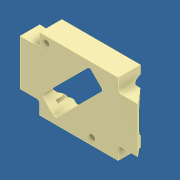
# Autodesk Inventor part: GuideCarotte
Saved by Autodesk Inventor 2018 (Build 220112000, 112)
## iProperties
Created: 2022-03-08
Part Number: GuideCarotte
Material: Nylon 6/6
Document SubType Name: Modeling
Designer: Nathann
Density: 1.13 g/cm^3
Appearance: Nylon 6
Mass: 63.4787 g
Surface Area: 154.903 cm^2
Volume: 56.1759 cm^3
Author: Nathann
Autodesk Inventor part; units mm, degrees
ref_plane "YZ Plane" through (0, 0, 0) normal (1, 0, 0) x (0, 1, 0)
ref_plane "XZ Plane" through (0, 0, 0) normal (0, 1, 0) x (-1, 0, 0)
sketch "Sketch24" plane through (0, 0, 0) normal (0, 1, 0) x (-1, 0, 0)
  line L0 (0, 0) -> (90, 0)
  line L1 (90, 0) -> (90, 55)
  line L2 (90, 55) -> (0, 55)
  line L3 (0, 55) -> (0, 0)
  dimension "d160" = 55
  dimension "d161" = 90
  constraints: 8 end point, 2 parallel, 1 horizontal, 1 perpendicular
  measures "d160" distance of L0.end L1.end
  measures "d161" distance of L1.end L2.end
extrude "Extrusion21" add sketch "Sketch24" along normal blind 17
sketch "Sketch25" plane through (0, 0, 0) normal (0, -1, 0) x (1, 0, 0)
  circle A0 centre (-70, 50) radius 2.5
  circle A1 centre (-35, 5) radius 2.5
  line L0 (0, 0) -> (-90, 0) projected
  line L1 (-90, 55) -> (0, 55) projected
  line L2 (-90, 0) -> (-90, 55) projected
  dimension "d164" = 5
  dimension "d165" = 5
  dimension "d166" = 5
  dimension "d167" = 5
  dimension "d168" = 20
  dimension "d169" = 55
  constraints: 2 centre point
  measures "d164" diameter of A0
  measures "d165" diameter of A1
  measures "d166" distance from line of L0 A1.centre
  measures "d167" distance from line of L1 A0.centre
  measures "d168" distance from line of L2 A0.centre
  measures "d169" distance from line of L2 A1.centre
extrude "Extrusion22" cut sketch "Sketch25" against normal blind 14
sketch "Sketch26" plane through (0, 17, 0) normal (0, 1, 0) x (1, 0, 0)
  line L0 (-63.0815, -3.8119) -> (-26.3119, -40.5815)
  line L1 (-26.3119, -40.5815) -> (-36.9185, -51.1881)
  line L2 (-36.9185, -51.1881) -> (-73.6881, -14.4185)
  line L3 (-73.6881, -14.4185) -> (-63.0815, -3.8119)
  line L4 (-90, 0) -> (-90, -55) projected
  line L5 (0, 0) -> (-90, 0) projected
  point P0 (0, -22.5)
  dimension "d172" = 15
  dimension "d173" = 52
  dimension "d176" = 47.3762
  dimension "d177" = 47.3762
  dimension "d181" = 16.3119
  dimension "d182" = 45
  dimension "d183" = 3.8119
  constraints: 8 end point, 3 perpendicular
  measures "d172" distance of L0.end L1.end
  measures "d173" distance of L1.end L2.end
  measures "d176" horizontal distance of L2.end L0.end
  measures "d177" vertical distance of L1.end L0.start
  measures "d181" distance from line of L4 L2.end
  measures "d182" angle of L4 L2
  measures "d183" distance from line of L5 L0.start
extrude "Extrusion23" cut sketch "Sketch26" against normal through all
ref_plane "Work Plane2" through (0, 0, 55) normal (0.9994, 0, 0.0349) x (0, 1, 0)
sketch "Sketch28" plane through (0, 0, 55) normal (0.9994, 0, 0.0349) x (0, 1, 0)
  circle A0 centre (27, -25.9665) radius 22.5
  line L0 (17, 0) -> (17, -54.9665) projected
  line L1 (0, -54.9665) -> (17, -54.9665) projected
  line L2 (0, 0) -> (0, -54.9665) projected
  dimension "d187" = 45
  dimension "d192" = 29
  dimension "d194" = 27
  constraints: 1 centre point
  measures "d187" diameter of A0
  measures "d192" distance from line of A0.centre L1
  measures "d194" distance from line of L2 A0.centre
extrude "Extrusion24" cut sketch "Sketch28" against normal through all
sketch "Sketch29" plane through (0, 17, 0) normal (0, 1, 0) x (1, 0, 0)
  line L0 (-26.3119, -40.5815) -> (-63.0815, -3.8119) projected
  line L1 (-44.6967, -22.1967) -> (-55.3033, -32.8033)
  line L2 (-73.6881, -14.4185) -> (-40.3293, -47.7773) projected
  arc A0 (-68.4344, -7.51) -> (-69.99, -9.0656) centre (-70.0818, -7.4182) ccw
  line L3 (-63.5547, -12.3896) -> (-68.4344, -7.51)
  line L4 (-69.99, -9.0656) -> (-65.1104, -13.9453)
  line L5 (-65.1104, -13.9453) -> (-63.5547, -12.3896)
  line L6 (-65.8208, -6.5512) -> (-63.0815, -3.8119) projected
  arc A1 (-31.5656, -47.49) -> (-30.01, -45.9344) centre (-29.9182, -47.5818) ccw
  line L7 (-34.8896, -41.0547) -> (-30.01, -45.9344)
  line L8 (-31.5656, -47.49) -> (-36.4453, -42.6104)
  line L9 (-36.4453, -42.6104) -> (-34.8896, -41.0547)
  line L10 (-29.0512, -43.3208) -> (-26.3119, -40.5815)
  point P0 (0, 0)
  point P1 (-73.6881, -14.4185)
  point P2 (-56.553, -49.6596)
  point P3 (-21.3119, -14.4185)
  point P4 (-40.3293, -47.7773)
  point P5 (-36.9185, -51.1881)
  dimension "d216" = 2.2
  dimension "d217" = 1.1
  dimension "d218" = 3.3
  dimension "d219" = 2.4
  dimension "d221" = 7.5
  dimension "d222" = 15
  constraints: 16 end point, 7 symmetric about line, 4 point on circle, 2 centre point, 1 midpoint, 1 parallel, 1 perpendicular, 3 other
  measures "d216" distance of L4.end L3.start
  measures "d217" distance from line of L3 A0.centre
  measures "d218" diameter of A0
  measures "d219" distance from line of A0.centre L6
  measures "d221" distance from line of A0.centre L0
extrude "Extrusion25" cut sketch "Sketch29" against normal blind 10.5
fillet "Fillet4" radius 2 4 edges at (-26.3119, 4.1375, 40.5815) (-63.0815, 8.5, 3.8119) (-73.6881, 3.9894, 14.4185) (-36.9185, 8.5, 51.1881)
sketch "Sketch31" plane through (0, 0, 0) normal (0, -1, 0) x (1, 0, 0)
  line L0 (7.4187, -6.4354) -> (-15, -6.4354)
  line L1 (-15, -6.4354) -> (-15, 10)
  line L2 (-15, 10) -> (7.4187, 10)
  line L3 (7.4187, 10) -> (7.4187, -6.4354)
  line L4 (0, 55) -> (0, 0) projected
  line L5 (0, 0) -> (-90, 0) projected
  line L6 (0, 0) -> (-90, 0) projected
  line L7 (-90, 55) -> (0, 55) projected
  line L8 (0, 27.5) -> (-90, 27.5)
  line L9 (-45, 62.4242) -> (-45, -8.4375)
  line L10 (-90, 0) -> (-90, 55) projected
  line L11 (7.4187, 61.4354) -> (-15, 61.4354)
  line L12 (-15, 61.4354) -> (-15, 45)
  line L13 (-15, 45) -> (7.4187, 45)
  line L14 (7.4187, 45) -> (7.4187, 61.4354)
  line L15 (-97.4187, -6.4354) -> (-75, -6.4354)
  line L16 (-75, -6.4354) -> (-75, 10)
  line L17 (-75, 10) -> (-97.4187, 10)
  line L18 (-97.4187, 10) -> (-97.4187, -6.4354)
  line L19 (-90, 55) -> (-90, 0)
  line L20 (-97.4187, 61.4354) -> (-75, 61.4354)
  line L21 (-75, 61.4354) -> (-75, 45)
  line L22 (-75, 45) -> (-97.4187, 45)
  line L23 (-97.4187, 45) -> (-97.4187, 61.4354)
  point P0 (-17, 0)
  point P1 (-17, 55)
  point P2 (-73, 0)
  point P3 (-73, 55)
  dimension "d227" = 15
  dimension "d228" = 10
  dimension "d229" = 45
  dimension "d230" = 90
  constraints: 38 end point, 14 symmetric about line, 3 perpendicular, 2 horizontal, 2 parallel, 1 midpoint, 1 vertical
  measures "d227" distance between parallel lines of L1 L4
  measures "d228" distance between parallel lines of L2 L5
  measures "d229" distance between parallel lines of L10 L9
  measures "d230" distance between parallel lines of L10 L4
extrude "Extrusion27" cut sketch "Sketch31" against normal through all contours L0 L1 L5 L4 L2 L3 | L1 L2 L4 L5 | L16 L15 L18 L17 L10 L5 | L5 L10 L17 L16 | L13 L12 L7 L4 | L4 L7 L12 L11 L14 L13 | L22 L23 L20 L21 L7 L10 | L10 L7 L21 L22
fillet "Fillet5" radius 2 4 edges at (-15, 7.0843, 10) (-75, 5.7918, 10) (-75, 7.1624, 45) (-15, 5.8494, 45)
sketch "Sketch32" plane through (0, 0, 45) normal (0, 0, 1) x (1, 0, 0)
  line L0 (0, 0) -> (-24.7878, 29.541)
  line L1 (-24.7878, 29.541) -> (8.6873, 22.432)
  line L2 (8.6873, 22.432) -> (0, 0)
  line L3 (0, 0) -> (-13, 0) projected
  dimension "d234" = 50
  constraints: 6 end point
  measures "d234" angle of L3 L0
extrude "Extrusion28" cut sketch "Sketch32" against normal through all
body "Solid2"
